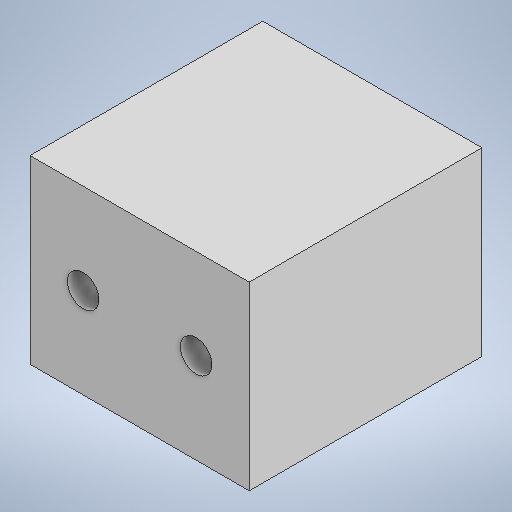
# Autodesk Inventor part: Honigschleuder_Steuerung_Netzteil_Notausklemme
Saved by Autodesk Inventor 2025 (Build 290162010, 162A)
## iProperties
Created: 2025-12-07
Part Number: Honigschleuder_Steuerung_Netzteil_Notausklemme
Material: Generisch
Document SubType Name: Modeling
Designer: max-h
Density: 1 g/cm^3
Appearance: Vorgabe
Author: max-h
Autodesk Inventor part; units mm, degrees
ref_plane "YZ Plane" through (0, 0, 0) normal (1, 0, 0) x (0, 1, 0)
ref_plane "XZ Plane" through (0, 0, 0) normal (0, 1, 0) x (-1, 0, 0)
ref_plane "XY Plane" through (0, 0, 0) normal (0, 0, 1) x (1, 0, 0)
sketch "Skizze1" plane through (0, 0, 0) normal (0, 1, 0) x (-1, 0, 0)
  line L0 (7.05, 5.0464) -> (-2.65, 5.0464)
  line L1 (-2.65, 5.0464) -> (-2.65, -5.2536)
  line L2 (-2.65, -5.2536) -> (7.05, -5.2536)
  line L3 (7.05, -5.2536) -> (7.05, 5.0464)
  point P0 (0, 0)
  dimension "d0" = 9.7
  dimension "d1" = 10.3
  constraints: 8 end point, 2 parallel, 1 horizontal, 1 perpendicular
  measures "d0" distance of L0.start L0.end
  measures "d1" distance of L2.end L0.start
extrude "Extrusion1" add sketch "Skizze1" along normal blind 8
sketch "Skizze2" plane through (-7.05, 0, 5.0464) normal (0, 0, 1) x (1, 0, 0)
  circle A0 centre (2.35, 4) radius 0.7
  circle A1 centre (7.35, 4) radius 0.7
  line L0 (0, 8) -> (9.7, 8) projected
  line L1 (2.35, 4) -> (7.35, 4) construction
  line L2 (0, 0) -> (0, 8) construction
  point P0 (7.05, 0)
  dimension "d4" = 4
  dimension "d5" = 5
  dimension "d6" = 2.35
  dimension "d7" = 1.4
  constraints: 2 centre point, 2 end point, 1 equal radius, 1 parallel
  measures "d4" distance from line of L0 L1.start
  measures "d5" distance of L1.start L1.end
  measures "d6" distance from line of L2 L1.start
  measures "d7" diameter of A0
extrude "Extrusion2" cut sketch "Skizze2" against normal blind 4
